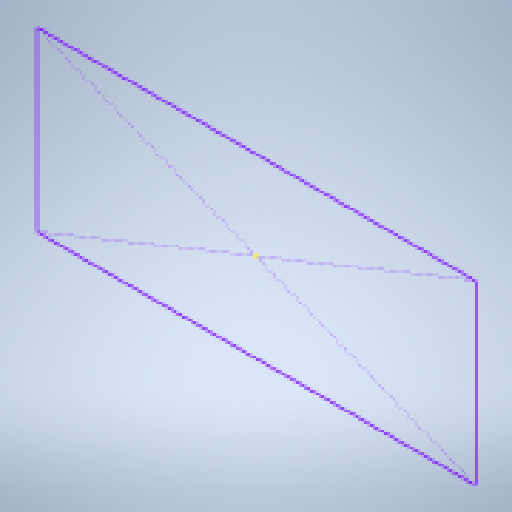
# Autodesk Inventor part: Sleeve
Saved by Autodesk Inventor 2023.2 (Build 272271000, 271)
## iProperties
Created: 2024-01-21
Part Number: Sleeve
Material: Nylon 6/6
Document SubType Name: Modeling
Designer: Nathan Cai
Density: 1.13 g/cm^3
Appearance: Nylon 6
Author: Nathan Cai
Autodesk Inventor part; units mm, degrees
ref_plane "YZ Plane" through (0, 0, 0) normal (1, 0, 0) x (0, 1, 0)
ref_plane "XZ Plane" through (0, 0, 0) normal (0, 1, 0) x (-1, 0, 0)
ref_plane "XY Plane" through (0, 0, 0) normal (0, 0, 1) x (1, 0, 0)
sketch "Sketch1" plane through (0, 0, 0) normal (0, 0, 1) x (1, 0, 0)
  line L0 (-15, -5) -> (15, -5)
  line L1 (15, -5) -> (15, 5)
  line L2 (15, 5) -> (-15, 5)
  line L3 (-15, 5) -> (-15, -5)
  line L4 (-15, -5) -> (15, 5) construction
  line L5 (15, -5) -> (-15, 5) construction
  line L6 (-17, 7) -> (17, 7)
  line L7 (17, 7) -> (17, -7)
  line L8 (17, -7) -> (-17, -7)
  line L9 (-17, -7) -> (-17, 7)
  line L10 (-15, 0) -> (-8.5, 0) construction
  line L11 (-8.5, 0) -> (-4.7776, -8.5875) construction
  circle A0 centre (-13.2482, 10.9542) radius 1.5875
  circle A1 centre (-13.2482, 10.9542) radius 3
  line L12 (-13.2482, 10.9542) -> (-19.3708, 3.6576) construction
  line L13 (-19.3708, 3.6576) -> (-4.7776, -8.5875) construction
  circle A2 centre (-4.7776, -8.5875) radius 1.5875
  circle A3 centre (-4.7776, -8.5875) radius 3
  point P0 (0, 0)
  point P1 (-2.2321, -7)
  point P2 (-9.2647, 7)
  point P3 (-13.8861, 7)
  point P4 (-7.3232, -7)
  dimension "d0" = 10
  dimension "d1" = 30
  dimension "d2" = 2
  dimension "d3" = 6.5
  dimension "d8" = 3.175
  dimension "d9" = 6
  dimension "d10" = 9.525
  dimension "d11" = 19.05
  dimension "d12" = 3.175
  dimension "d13" = 6
  dimension "d14" = 40
  constraints: 27 end point, 4 centre point, 3 coincident, 3 horizontal, 3 midpoint, 3 parallel, 2 perpendicular, 1 point on line, 1 vertical, 7 other
  measures "d0" distance between parallel lines of L0 L2
  measures "d1" distance between parallel lines of L3 L1
  measures "d2" distance between parallel lines of L2 L6
  measures "d3" distance of L10.start L10.end
  measures "d8" diameter of A0
  measures "d9" diameter of A1
  measures "d10" distance from line of L13 A0.centre
  measures "d11" distance from line of L11.end L12
  measures "d12" diameter of A2
  measures "d13" diameter of A3
  measures "d14" angle of L0 L13
extrude "Extrusion1" add sketch "Sketch1" along normal blind 31 contours L6 L7 L8 A3 L9 | A3 L8 | L8 A3
fillet "Fillet1" radius 4 2 edges at (-2.2321, -7, 15.5) (-7.3232, -7, 15.5)
sketch "Sketch2" plane through (0, 0, 0) normal (0, 0, -1) x (-1, 0, 0)
  line L0 (-22.5, -0.875) -> (22.5, -0.875)
  line L1 (22.5, -0.875) -> (22.5, 0.875)
  line L2 (22.5, 0.875) -> (-22.5, 0.875)
  line L3 (-22.5, 0.875) -> (-22.5, -0.875)
  line L4 (-22.5, -0.875) -> (22.5, 0.875) construction
  line L5 (22.5, -0.875) -> (-22.5, 0.875) construction
  point P0 (0, 0)
  dimension "d18" = 45
  dimension "d19" = 1.75
  constraints: 12 end point, 2 midpoint, 2 parallel, 1 horizontal, 1 perpendicular
  measures "d18" distance of L2.end L1.end
  measures "d19" distance of L1.end L0.end
extrude "Extrusion2" cut sketch "Sketch2" against normal blind 8
fillet "Fillet2" radius 3.5 1 edges at (-17, -7, 15.5)
body "Solid1"
